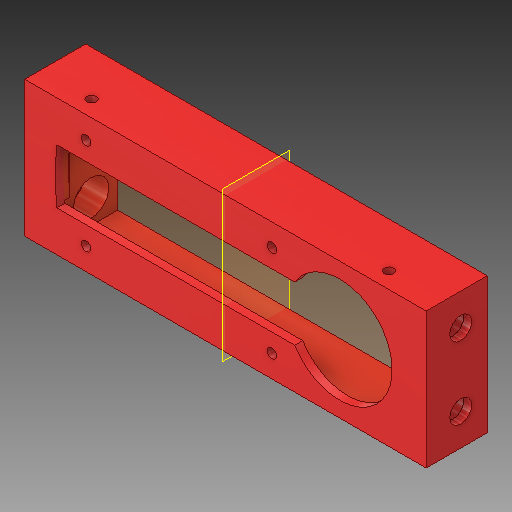
# Autodesk Inventor part: Syringe Pump Holder
Saved by Autodesk Inventor 2018.1 (Build 221171000, 171)
## iProperties
Created: 2024-06-06
Part Number: Syringe Pump Holder
Material: Generic
Document SubType Name: Modeling
Designer: Enrico
Density: 1 g/cm^3
Appearance: Light Red
Author: Enrico
Autodesk Inventor part; units mm, degrees
ref_plane "YZ Plane" through (0, 0, 0) normal (1, 0, 0) x (0, 1, 0)
ref_plane "XZ Plane" through (0, 0, 0) normal (0, 1, 0) x (-1, 0, 0)
ref_plane "Work Plane1" through (0, 0, 0.1) normal (0, 0, 1) x (1, 0, 0)
sketch "Sketch1" plane through (0, 0, 0.1) normal (0, 0, 1) x (1, 0, 0)
  circle A0 centre (-52.5, -39.75) radius 1.5 projected
  circle A1 centre (17.5, -5.25) radius 1.5 projected
  circle A2 centre (-52.5, -5.25) radius 1.5 projected
  circle A3 centre (17.5, -39.75) radius 1.5 projected
  line L0 (-62.5, -18) -> (-24, -18) projected
  line L1 (-24, -18) -> (-24, -27) projected
  line L2 (-24, -27) -> (-62.5, -27) projected
  line L3 (-62.5, -44) -> (-62.5, -27) construction
  line L4 (62.5, -44) -> (-62.5, -44) construction
  line L5 (62.5, -22.5) -> (62.5, -44) construction
  circle A4 centre (43, -22.5) radius 19.5 projected
  line L6 (62.5, -1) -> (62.5, -22.5) construction
  line L7 (-62.5, -1) -> (62.5, -1) construction
  line L8 (-62.5, -18) -> (-62.5, -1) construction
  circle A5 centre (43, -22.5) radius 19.8
  line L9 (23.5, -12.5) -> (-24, -12.5)
  line L10 (23.5, -32.5) -> (-24, -32.5)
  line L11 (23.5, -12.2) -> (-24, -12.2)
  line L12 (23.5, -32.8) -> (-24, -32.8)
  line L13 (-63.5, 0) -> (-63.5, -45) projected
  line L14 (63.5, 0) -> (-63.5, 0) projected
  line L15 (-63.5, -45) -> (63.5, -45) projected
  line L16 (63.5, -45) -> (63.5, 0) projected
  line L17 (66.6, -48.1) -> (-66.6, -48.1)
  line L18 (-66.6, -48.1) -> (-66.6, 3.1)
  line L19 (-66.6, 3.1) -> (66.6, 3.1)
  line L20 (66.6, 3.1) -> (66.6, -48.1)
  circle A6 centre (17.5, -39.75) radius 1.8
  circle A7 centre (17.5, -5.25) radius 1.8
  circle A8 centre (-52.5, -39.75) radius 1.8
  circle A9 centre (-52.5, -5.25) radius 1.8
  line L21 (23.5, -32.8) -> (26.0899, -32.8)
  line L22 (23.5, -12.2) -> (26.0899, -12.2)
  line L23 (-24, -12.2) -> (-63.5, -12.2)
  line L24 (-24, -32.8) -> (-63.5, -32.8)
  point P0 (0, 0)
  dimension "d0" = 0.3
  dimension "d1" = 0.3
  dimension "d2" = 0.3
  dimension "d3" = 3.1
  dimension "d4" = 0.3
  dimension "d5" = 0.3
  dimension "d6" = 0.3
  dimension "d7" = 0.3
  constraints: 24 end point, 5 centre point, 3 horizontal, 3 parallel, 3 point on line, 2 point on circle, 1 collinear, 1 horizontal alignment, 7 other
  measures "d1" distance between parallel lines of L9 L11
  measures "d2" distance between parallel lines of L10 L12
  measures "d3" distance between parallel lines of L15 L17
  measures "d4" radial gap between concentric circles of A3 A6
  measures "d5" radial gap between concentric circles of A1 A7
  measures "d6" radial gap between concentric circles of A0 A8
  measures "d7" radial gap between concentric circles of A2 A9
extrude "Extrusion1" add sketch "Sketch1" along normal blind 3 contours A5 L22 L11 L23 L13 L14 L16 L15 L24 L12 L21 | L17 L18 L19 L20
sketch "Sketch2" plane through (0, 0, 0.1) normal (0, 0, -1) x (-1, 0, 0)
  circle A0 centre (52.5, -5.25) radius 1.8 construction
  circle A1 centre (52.5, -39.75) radius 1.8 construction
  circle A2 centre (-17.5, -5.25) radius 1.8 construction
  circle A3 centre (-17.5, -39.75) radius 1.8 construction
  line L0 (-66.6, -48.1) -> (66.6, -48.1) projected
  line L1 (66.6, -48.1) -> (66.6, 3.1) projected
  line L2 (66.6, 3.1) -> (-66.6, 3.1) projected
  line L3 (-66.6, 3.1) -> (-66.6, -48.1) projected
  line L4 (-26.0899, -12.2) -> (63.5, -12.2) construction
  line L5 (63.5, -12.2) -> (63.5, -32.8) construction
  line L6 (63.5, -32.8) -> (-26.0899, -32.8) construction
  arc A4 (-26.0899, -12.2) -> (-26.0899, -32.8) centre (-43, -22.5) ccw construction
  line L7 (-63.6, 0.1) -> (63.6, 0.1)
  line L8 (63.6, 0.1) -> (63.6, -45.1)
  line L9 (63.6, -45.1) -> (-63.6, -45.1)
  line L10 (-63.6, -45.1) -> (-63.6, 0.1)
  point P0 (0, 0)
  dimension "d10" = 3
  constraints: 8 end point, 3 other
  measures "d10" distance between parallel lines of L2 L7
extrude "Extrusion2" add sketch "Sketch2" along normal blind 20
sketch "Sketch3" plane through (-66.6, -48.1, 3.1) normal (0, -1, 0) x (1, 0, 0)
  line L0 (3.1, -4.1) -> (130.1, -4.1) construction
  line L1 (3.1, -119.3) -> (3.1, -4.1) projected
  line L2 (3.1, -119.3) -> (130.1, -119.3) projected
  line L3 (130.1, -4.1) -> (130.1, -119.3) projected
  circle A0 centre (122.1, -6.1) radius 1.5 construction
  circle A1 centre (10.1, -6.1) radius 1.5 construction
  circle A2 centre (10.1, -6.1) radius 1.8
  circle A3 centre (122.1, -6.1) radius 1.8
  point P0 (66.6, -3.1)
  dimension "d13" = 0.3
  dimension "d14" = 0.3
  constraints: 2 centre point
  measures "d13" radial gap between concentric circles of A1 A2
  measures "d14" radial gap between concentric circles of A0 A3
extrude "Extrusion3" cut sketch "Sketch3" against normal through all
sketch "Sketch4" plane through (-66.6, -48.1, 3.1) normal (-1, 0, 0) x (0, 0, 1)
  line L0 (-4.1, 3.1) -> (-4.1, 48.1) construction
  line L1 (-4.1, 3.1) -> (-119.3, 3.1) construction
  line L2 (-119.3, 3.1) -> (-119.3, 48.1) projected
  line L3 (-119.3, 48.1) -> (-4.1, 48.1) construction
  circle A0 centre (-6.1, 9.1) radius 1.5 construction
  circle A1 centre (-6.1, 42.1) radius 1.5 construction
  circle A2 centre (-13, 12) radius 6.65
  line L4 (0, 0) -> (-23, 0) projected
  line L5 (-23, 0) -> (-23, 51.2) projected
  line L6 (-23, 25.6) -> (0, 25.6) construction
  line L7 (0, 15.3) -> (0, 35.9) projected
  circle A3 centre (-13, 39.2) radius 6.65
  point P0 (-3.1, 48.1)
  dimension "d17" = 13.3
  dimension "d18" = 12
  dimension "d19" = 10
  constraints: 2 centre point, 2 end point, 2 midpoint, 1 symmetric about line, 1 other
  measures "d17" diameter of A2
  measures "d18" distance from line of L4 A2.centre
  measures "d19" distance from line of L5 A2.centre
extrude "Extrusion4" cut sketch "Sketch4" against normal through all
sketch "Sketch5" plane through (-66.6, -48.1, 3.1) normal (-1, 0, 0) x (0, 0, 1)
  circle A0 centre (-13, 12) radius 6.65 projected
  circle A1 centre (-13, 39.2) radius 6.65 projected
  line L0 (0, 0) -> (-23, 0) projected
  line L1 (0, 51.2) -> (0, 0) projected
  line L2 (0, 51.2) -> (-23, 51.2) projected
  line L3 (-23, 0) -> (-23, 51.2) projected
  point P0 (-3.1, 48.1)
extrude "Extrusion5" add sketch "Sketch5" along normal blind 6
sketch "Sketch6" plane through (-72.6, -48.1, 3.1) normal (-1, 0, 0) x (0, 0, 1)
  circle A0 centre (-13, 39.2) radius 6.65 construction
  circle A1 centre (-13, 12) radius 6.65 construction
  line L0 (-23, 0) -> (0, 0) projected
  line L1 (0, 0) -> (0, 51.2) projected
  line L2 (0, 51.2) -> (-23, 51.2) projected
  line L3 (-23, 51.2) -> (-23, 0) projected
  circle A2 centre (-13, 12) radius 4.15
  circle A3 centre (-13, 39.2) radius 4.15
  point P0 (-3.1, 48.1)
  dimension "d24" = 8.3
  dimension "d25" = 8.3
  constraints: 2 centre point, 2 coincident
  measures "d24" diameter of A2
  measures "d25" diameter of A3
extrude "Extrusion6" add sketch "Sketch6" along normal blind 3
ref_plane "Work Plane2" through (0, -45.1, 0.1) normal (1, 0, 0) x (0, 0, -1)
mirror "Mirror1" about plane through (0, -45.1, 0.1) normal (1, 0, 0) of "Extrusion5", "Extrusion6"
ref_plane "Work Plane3" through (-63.5, -27, 0) normal (0, 0, -1) x (0, 1, 0)
sketch "Sketch7" plane through (0, 0, 3.1) normal (0, 0, 1) x (1, 0, 0)
  circle A0 centre (-52.5, -5.25) radius 1.8 projected
  circle A1 centre (-52.5, -39.75) radius 1.8 projected
  circle A2 centre (17.5, -5.25) radius 1.8 projected
  circle A3 centre (17.5, -39.75) radius 1.8 projected
  line L0 (75.6, -48.1) -> (-75.6, -48.1) projected
  line L1 (75.6, -48.1) -> (75.6, 3.1) projected
  line L2 (-75.6, 3.1) -> (75.6, 3.1) projected
  line L3 (-75.6, -48.1) -> (-75.6, 3.1) projected
  line L4 (26.0899, -32.8) -> (-63.5, -32.8) projected
  line L5 (-63.5, -32.8) -> (-63.5, -12.2) projected
  line L6 (-63.5, -12.2) -> (26.0899, -12.2) projected
  arc A4 (26.0899, -32.8) -> (26.0899, -12.2) centre (43, -22.5) ccw projected
  line L7 (-63.5, -12.2) -> (-63.5, -32.8) projected
  line L8 (-63.6, 0.1) -> (-63.6, -45.1) construction
  arc A5 (-63.5, -12.2) -> (-63.5, -32.8) centre (24.6083, -22.5) ccw
  point P0 (0, 0)
  point P1 (-63.6, -22.5)
  point P2 (-64.1, -22.5)
  dimension "d28" = 0.5
  constraints: 3 point on circle, 1 centre point, 1 horizontal alignment, 1 midpoint
  measures "d28" distance from line of L8 point (-64.1, -22.5)
extrude "Extrusion7" cut sketch "Sketch7" against normal blind 5 contours A5 L5
body "Solid1"
